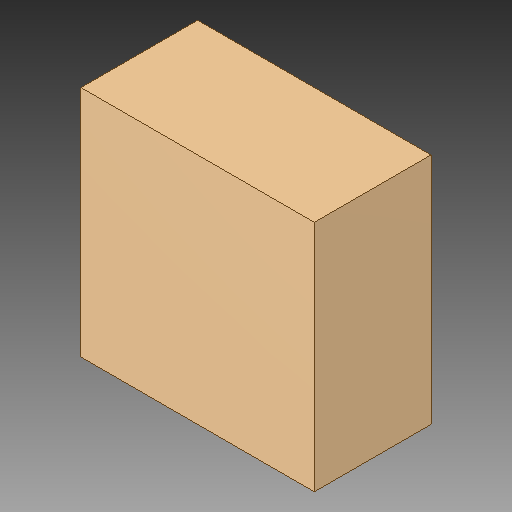
# Autodesk Inventor part: SMD_PHOTORESISTOR_5MM
Saved by Autodesk Inventor 2017 (Build 210142000, 142)
## iProperties
Created: 2019-06-13
Part Number: SMD_PHOTORESISTOR_5MM
Material: Generic
Document SubType Name: Modeling
Designer: Marc
Density: 1 g/cm^3
Appearance: SMD_PHOTORESISTOR_5MM, SMD_PHOTORESISTOR_5MM
Author: Marc
Autodesk Inventor part; units mm, degrees
ref_plane "YZ Plane" through (0, 0, 0) normal (1, 0, 0) x (0, 1, 0)
ref_plane "XZ Plane" through (0, 0, 0) normal (0, 1, 0) x (-1, 0, 0)
ref_plane "XY Plane" through (0, 0, 0) normal (0, 0, 1) x (1, 0, 0)
sketch "SMD_PHOTORESISTOR_5MM, SMD_PHOTORESISTOR_5MM_70" plane through (0, 0, 0) normal (0, 0, 1) x (1, 0, 0)
  line L0 (1, -1) -> (-1, -1)
  line L1 (-1, -1) -> (-1, 1)
  line L2 (-1, 1) -> (1, 1)
  line L3 (1, 1) -> (1, -1)
  constraints: 8 end point
extrude "Extrusion1" add sketch "SMD_PHOTORESISTOR_5MM, SMD_PHOTORESISTOR_5MM_70" along normal blind 1
body "Solid1"
